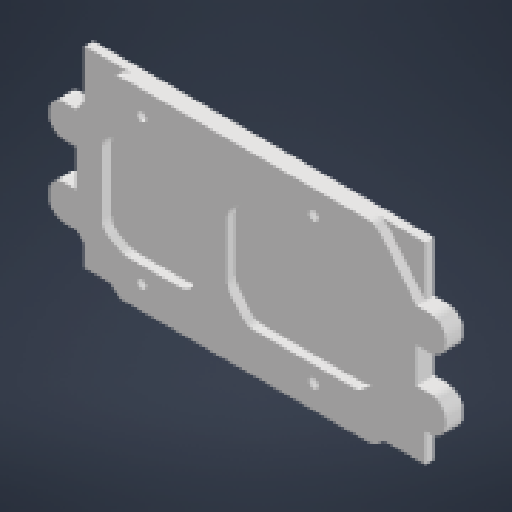
# Autodesk Inventor part: Pi_holder
Saved by Autodesk Inventor 2026.1 (Build 301233020, 233B)
## iProperties
Created: 2025-10-27
Part Number: Pi_holder
Material: Generic
Document SubType Name: Modeling
Designer: Mikke
Density: 1 g/cm^3
Appearance: Default
Author: Mikke
Autodesk Inventor part; units mm, degrees
ref_plane "YZ Plane" through (0, 0, 0) normal (1, 0, 0) x (0, 1, 0)
ref_plane "XZ Plane" through (0, 0, 0) normal (0, 1, 0) x (-1, 0, 0)
ref_plane "XY Plane" through (0, 0, 0) normal (0, 0, 1) x (1, 0, 0)
sketch "Sketch1" plane through (0, 0, 0) normal (0, 0, 1) x (1, 0, 0)
  line L0 (-3.3178, 34.6574) -> (-118.4066, 34.6574)
  line L1 (-118.4066, 34.6574) -> (-118.4066, -30.3526)
  line L2 (-118.4066, -30.3526) -> (-3.3178, -30.3526)
  line L3 (-3.3178, -30.3526) -> (-3.3178, 34.6574)
  line L4 (-118.4066, 17.6954) -> (-127.435, 17.6954)
  line L5 (-127.435, 17.6954) -> (-127.435, 6.6388)
  line L6 (-127.435, 6.6388) -> (-118.4066, 6.6388)
  line L7 (-118.4066, 6.6388) -> (-118.4066, 17.6954)
  line L8 (-118.4066, -17.6281) -> (-127.435, -17.6281)
  line L9 (-127.435, -17.6281) -> (-127.435, -5.7358)
  line L10 (-127.435, -5.7358) -> (-118.4066, -5.7358)
  line L11 (-118.4066, -5.7358) -> (-118.4066, -17.6281)
  line L12 (-3.3178, -17.6281) -> (6.4307, -17.6281)
  line L13 (6.4307, -17.6281) -> (6.4307, -5.7358)
  line L14 (6.4307, -5.7358) -> (-3.3178, -5.7358)
  line L15 (-3.3178, -5.7358) -> (-3.3178, -17.6281)
  line L16 (-3.3178, 17.6954) -> (6.4307, 17.6954)
  line L17 (6.4307, 17.6954) -> (6.4307, 6.1817)
  line L18 (6.4307, 6.1817) -> (-3.3178, 6.1817)
  line L19 (-3.3178, 6.1817) -> (-3.3178, 17.6954)
  point P0 (0, 0)
  point P1 (-3.3178, -5.7358)
  point P2 (-3.3178, 6.1817)
  constraints: 40 end point, 10 parallel, 9 point on line, 5 horizontal, 5 perpendicular
extrude "Extrusion1" add sketch "Sketch1" along normal blind 6
sketch "Sketch2" plane through (0, 0, 6) normal (0, 0, 1) x (1, 0, 0)
  circle A0 centre (-38.1293, 26.639) radius 1.5 projected
  circle A1 centre (-38.1293, -22.361) radius 1.5 projected
  circle A2 centre (-96.1293, -22.361) radius 1.5 projected
  circle A3 centre (-96.1293, 26.639) radius 1.5 projected
  line L0 (6.4307, 17.6954) -> (-3.3178, 17.6954) projected
  line L1 (-3.3178, 17.6954) -> (-3.3178, 34.6574) projected
  line L2 (-3.3178, 34.6574) -> (-118.4066, 34.6574) projected
  line L3 (-118.4066, 34.6574) -> (-118.4066, 17.6954) projected
  line L4 (-118.4066, 17.6954) -> (-127.435, 17.6954) projected
  line L5 (-127.435, 17.6954) -> (-127.435, 6.6388) projected
  line L6 (-127.435, 6.6388) -> (-118.4066, 6.6388) projected
  line L7 (-118.4066, 6.6388) -> (-118.4066, -5.7358) projected
  line L8 (-118.4066, -5.7358) -> (-127.435, -5.7358) projected
  line L9 (-127.435, -5.7358) -> (-127.435, -17.6281) projected
  line L10 (-127.435, -17.6281) -> (-118.4066, -17.6281) projected
  line L11 (-118.4066, -17.6281) -> (-118.4066, -30.3526) projected
  line L12 (-118.4066, -30.3526) -> (-3.3178, -30.3526) projected
  line L13 (-3.3178, -30.3526) -> (-3.3178, -17.6281) projected
  line L14 (-3.3178, -17.6281) -> (6.4307, -17.6281) projected
  line L15 (6.4307, -17.6281) -> (6.4307, -5.7358) projected
  line L16 (6.4307, -5.7358) -> (-3.3178, -5.7358) projected
  line L17 (-3.3178, -5.7358) -> (-3.3178, 6.1817) projected
  line L18 (-3.3178, 6.1817) -> (6.4307, 6.1817) projected
  line L19 (6.4307, 6.1817) -> (6.4307, 17.6954) projected
  circle A4 centre (-96.1293, 26.639) radius 2
  circle A5 centre (-96.1293, -22.361) radius 2
  circle A6 centre (-38.1293, -22.361) radius 2
  circle A7 centre (-38.1293, 26.639) radius 2
  point P0 (0, 0)
  dimension "d9" = 4
  dimension "d10" = 4
  dimension "d11" = 4
  dimension "d12" = 4
  constraints: 4 centre point, 4 coincident
  measures "d9" diameter of A4
  measures "d10" diameter of A5
  measures "d11" diameter of A6
  measures "d12" diameter of A7
extrude "Extrusion2" cut sketch "Sketch2" against normal blind 6 contours A0 | A1 | A2 | A3 | A4 | A5 | A6 | A7
sketch "Sketch3" plane through (0, 0, 0) normal (0, 0, -1) x (-1, 0, 0)
  circle A0 centre (-1.5276, 12) radius 1.75 projected
  line L0 (-6.4307, 17.6954) -> (3.3178, 17.6954) projected
  line L1 (-6.4307, 6.1817) -> (-6.4307, 17.6954) projected
  line L2 (3.3178, 6.1817) -> (-6.4307, 6.1817) projected
  line L3 (3.3178, -5.7358) -> (3.3178, 6.1817) projected
  line L4 (-6.4307, -5.7358) -> (3.3178, -5.7358) projected
  line L5 (-6.4307, -17.6281) -> (-6.4307, -5.7358) projected
  line L6 (3.3178, -17.6281) -> (-6.4307, -17.6281) projected
  line L7 (3.3178, -30.3526) -> (3.3178, -17.6281) projected
  line L8 (118.4066, -30.3526) -> (3.3178, -30.3526) projected
  line L9 (118.4066, -17.6281) -> (118.4066, -30.3526) projected
  line L10 (127.435, -17.6281) -> (118.4066, -17.6281) projected
  line L11 (127.435, -5.7358) -> (127.435, -17.6281) projected
  line L12 (118.4066, -5.7358) -> (127.435, -5.7358) projected
  line L13 (118.4066, 6.6388) -> (118.4066, -5.7358) projected
  line L14 (127.435, 6.6388) -> (118.4066, 6.6388) projected
  line L15 (127.435, 17.6954) -> (127.435, 6.6388) projected
  line L16 (118.4066, 17.6954) -> (127.435, 17.6954) projected
  line L17 (118.4066, 34.6574) -> (118.4066, 17.6954) projected
  line L18 (3.3178, 34.6574) -> (118.4066, 34.6574) projected
  line L19 (3.3178, 17.6954) -> (3.3178, 34.6574) projected
  circle A1 centre (-1.5276, -12) radius 1.75 projected
  circle A2 centre (122.7276, -12) radius 1.75 projected
  circle A3 centre (122.7276, 12) radius 1.75 projected
  point P0 (0, 0)
extrude "Extrusion3" cut sketch "Sketch3" against normal blind 6 contours A0 | A1 | A2 | A3
sketch "Sketch4" plane through (0, 0, 6) normal (0, 0, 1) x (1, 0, 0)
  circle A0 centre (-38.1293, -22.361) radius 1.5 projected
  circle A1 centre (-96.1293, -22.361) radius 1.5 projected
  circle A2 centre (-38.1293, 26.639) radius 1.5 projected
  circle A3 centre (-96.1293, 26.639) radius 1.5 projected
  arc A4 (-108.1293, -22.361) -> (-100.1293, -30.361) centre (-100.1293, -22.361) ccw projected
  line L0 (-108.1293, 26.639) -> (-108.1293, -22.361) projected
  arc A5 (-100.1293, 34.639) -> (-108.1293, 26.639) centre (-100.1293, 26.639) ccw projected
  line L1 (-21.1293, 34.639) -> (-100.1293, 34.639) projected
  arc A6 (-13.1293, 26.639) -> (-21.1293, 34.639) centre (-21.1293, 26.639) ccw projected
  line L2 (-13.1293, -22.361) -> (-13.1293, 26.639) projected
  arc A7 (-21.1293, -30.361) -> (-13.1293, -22.361) centre (-21.1293, -22.361) ccw projected
  line L3 (-100.1293, -30.361) -> (-21.1293, -30.361) projected
  line L4 (-127.435, -17.6281) -> (-118.4066, -17.6281) projected
  line L5 (-118.4066, -30.3526) -> (-3.3178, -30.3526) projected
  line L6 (-118.4066, 34.6574) -> (-118.4066, 17.6954) projected
  line L7 (-118.4066, 17.6954) -> (-104.664, 34.6574)
  line L8 (-3.3178, 34.6574) -> (-118.4066, 34.6574) projected
  line L9 (-3.3178, 17.6954) -> (-3.3178, 34.6574) projected
  line L10 (-3.3178, 17.6954) -> (-17.3486, 34.9264)
  line L11 (-3.3178, -17.6281) -> (6.4307, -17.6281) projected
  line L12 (-109.439, 13.3074) -> (-100.4496, 20.3827)
  line L13 (-100.4496, 20.3827) -> (-26.1151, 20.3827)
  line L14 (-26.1151, 20.3827) -> (-15.4724, 9.6699)
  line L15 (-15.4724, 9.6699) -> (-15.4724, -9.7854)
  line L16 (-15.4724, -9.7854) -> (-22.5627, -16.9004)
  line L17 (-22.5627, -16.9004) -> (-102.211, -16.9004)
  line L18 (-102.211, -16.9004) -> (-109.439, -13.1126)
  line L19 (-109.439, -13.1126) -> (-109.439, 13.3074)
  line L20 (-80.6051, 20.3827) -> (-74.943, 13.3074)
  line L21 (-74.943, 13.3074) -> (-74.943, -8.5904)
  line L22 (-74.943, -8.5904) -> (-80.6051, -16.9004)
  line L23 (-60.8622, 20.3827) -> (-67.4019, 13.1693)
  line L24 (-67.4019, 13.1693) -> (-67.4019, -8.7285)
  line L25 (-67.4019, -8.7285) -> (-60.8622, -16.9004)
  line L26 (-3.3178, -30.3526) -> (-3.3178, -17.6281) projected
  line L27 (-3.3178, -17.6281) -> (-17.6408, -30.3526)
  line L28 (-118.4066, -30.3526) -> (-3.3178, -30.3526) projected
  line L29 (-118.4066, -17.6281) -> (-103.6048, -30.3526)
  line L30 (-118.4066, -17.6281) -> (-118.4066, -30.3526) projected
  line L31 (-118.4066, -17.6281) -> (-118.4066, -30.3526)
  line L32 (-118.4066, -30.3526) -> (-103.6048, -30.3526)
  line L33 (-3.3178, -17.6281) -> (-3.3178, -30.3526)
  line L34 (-17.6408, -30.3526) -> (-3.3178, -30.3526)
  point P0 (0, 0)
  point P1 (-17.1296, 34.6574)
  point P2 (-17.6408, -30.3526)
  constraints: 44 end point, 7 point on line, 5 perpendicular, 2 collinear, 2 parallel, 1 horizontal, 1 vertical
extrude "Extrusion4" cut sketch "Sketch4" against normal blind 6 contours L27 L26 L5 | L5 L30 L29 | L18 L19 L12 L0 | L0 L12 L13 L20 L21 L22 L17 L18 | L25 L24 L23 L13 L14 L15 L16 L17 | L8 L7 L6 | L8 L9 L10
fillet "Fillet1" radius 5 28 edges at (-127.435, 17.6954, 3) (-127.435, 6.6388, 3) (-127.435, -5.7358, 3) (-127.435, -17.6281, 3) (-104.664, 34.6574, 3) (-17.1296, 34.6574, 3) (6.4307, 17.6954, 3) (6.4307, 6.1817, 3) (6.4307, -5.7358, 3) (6.4307, -17.6281, 3) (-17.6408, -30.3526, 3) (-103.6048, -30.3526, 3) (-80.6051, 20.3827, 3) (-74.943, 13.3074, 3) (-26.1151, 20.3827, 3) (-15.4724, 9.6699, 3) (-15.4724, -9.7854, 3) (-22.5627, -16.9004, 3) (-60.8622, 20.3827, 3) (-67.4019, 13.1693, 3) (-67.4019, -8.7285, 3) (-60.8622, -16.9004, 3) (-109.439, -13.1126, 3) (-102.211, -16.9004, 3) (-100.4496, 20.3827, 3) (-109.439, 13.3074, 3) (-74.943, -8.5904, 3) (-80.6051, -16.9004, 3)
body "Solid1"
